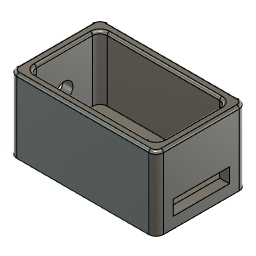
IIT Plant Watch v3 (Autodesk Fusion 360 design; units mm, degrees)
Autodesk Fusion 360 part; units mm, degrees
sketch "Sketch1" plane through (0, 0, 0) normal (0, 1, 0) x (1, 0, 0) in component "Box"
  line L0 (30, -18.5) -> (-30, -18.5)
  line L1 (-30, -18.5) -> (-30, 18.5)
  line L2 (-30, 18.5) -> (30, 18.5)
  line L3 (30, 18.5) -> (30, -18.5)
  line L4 (30, -18.5) -> (-30, 18.5) construction
  line L5 (-30, -18.5) -> (30, 18.5) construction
  dimension "d1" = 60
  dimension "d2" = 37
  constraint horizontal L0
  constraint perpendicular L0 L1
  constraint parallel L0 L2
  constraint parallel L1 L3
  constraint coincident L4 origin
  constraint coincident L5 origin
  measures "d1" distance of L1.end L2.end
  measures "d2" distance of L0.end L1.end
extrude "Extrude1" add sketch "Sketch1" along normal blind 30 in component "Box"
sketch "Sketch2" plane through (0, 30, 0) normal (0, 1, 0) x (-1, 0, 0) in component "Box"
  line L0 (-30, -18.5) -> (30, -18.5)
  line L1 (30, -18.5) -> (30, 18.5)
  line L2 (30, 18.5) -> (-30, 18.5)
  line L3 (-30, 18.5) -> (-30, -18.5)
  line L4 (26, -14.5) -> (26, 14.5)
  line L5 (26, 14.5) -> (-26, 14.5)
  line L6 (-26, 14.5) -> (-26, -14.5)
  line L7 (-26, -14.5) -> (26, -14.5)
  dimension "d5" = -4
extrude "Extrude2" cut sketch "Sketch2" against normal up to surface (26 mm away) contours L4 L5 L6 L7 in component "Box"
fillet "Fillet1" radius 3 4 edges at (26, 17, -14.5) (26, 17, 14.5) (-26, 17, -14.5) (-26, 17, 14.5) in component "Box"
fillet "Fillet2" radius 3 4 edges at (-30, 15, 18.5) (-30, 15, -18.5) (30, 15, 18.5) (30, 15, -18.5) in component "Box"
sketch "Sketch3" plane through (0, 0, 18.5) normal (0, 0, 1) x (1, 0, 0) in component "Box"
  line L0 (27, 0) -> (27, 30)
  line L1 (27, 30) -> (-27, 30)
  line L2 (-27, 30) -> (-27, 0)
  line L3 (-27, 0) -> (27, 0)
sketch "Sketch4" plane through (-30, 0, 0) normal (-1, 0, 0) x (0, 0, 1) in component "Box"
  line L0 (-15.5, 30) -> (-15.5, 0)
  line L1 (-15.5, 0) -> (15.5, 0)
  line L2 (15.5, 0) -> (15.5, 30)
  line L3 (15.5, 30) -> (-15.5, 30)
  circle A0 centre (0, 15) radius 3.5
  line L4 (-18.5, 30) -> (-18.5, 0)
  dimension "d12" = 7
  dimension "d13" = 18.5
  dimension "d14" = 15
  measures "d12" diameter of A0
  measures "d13" distance of A0.centre L4
  measures "d14" distance of L1 A0.centre
extrude "Extrude3" cut sketch "Sketch4" against normal up to surface (4 mm away) contours A0 in component "Box"
sketch "Sketch5" plane through (30, 0, 0) normal (1, 0, 0) x (0, 0, -1) in component "Box"
  line L0 (15.5, 0) -> (15.5, 30)
  line L1 (15.5, 30) -> (-15.5, 30)
  line L2 (-15.5, 30) -> (-15.5, 0)
  line L3 (-15.5, 0) -> (15.5, 0)
  line L4 (0, 0) -> (0, 36) construction
  line L5 (11.5, 4.5) -> (-11.5, 4.5)
  line L6 (-11.5, 4.5) -> (-11.5, 10.5)
  line L7 (-11.5, 10.5) -> (11.5, 10.5)
  line L8 (11.5, 10.5) -> (11.5, 4.5)
  line L9 (11.5, 4.5) -> (-11.5, 10.5) construction
  line L10 (-11.5, 4.5) -> (11.5, 10.5) construction
  point P0 (0, 7.5)
  dimension "d17" = 23
  dimension "d18" = 6
  dimension "d19" = 7.5
  constraint coincident L4.start origin
  constraint perpendicular L1 L4
  constraint horizontal L5
  constraint perpendicular L5 L6
  constraint parallel L5 L7
  constraint parallel L6 L8
  constraint coincident L9 P0
  constraint coincident L10 P0
  constraint coincident L4 P0
  measures "d17" distance of L6.end L7.end
  measures "d18" distance of L5.end L6.end
  measures "d19" distance of L3 P0
extrude "Extrude4" cut sketch "Sketch5" against normal up to surface (4 mm away) contours L5 L6 L7 L8 in component "Box"
sketch "Sketch6" plane through (0, 0, 0) normal (0, -1, 0) x (1, 0, 0) in component "Box"
  arc A0 (27, -18.5) -> (30, -15.5) centre (27, -15.5) ccw
  line L0 (30, -15.5) -> (30, 15.5)
  arc A1 (30, 15.5) -> (27, 18.5) centre (27, 15.5) ccw
  line L1 (27, 18.5) -> (-27, 18.5)
  arc A2 (-27, 18.5) -> (-30, 15.5) centre (-27, 15.5) ccw
  line L2 (-30, 15.5) -> (-30, -15.5)
  arc A3 (-30, -15.5) -> (-27, -18.5) centre (-27, -15.5) ccw
  line L3 (-27, -18.5) -> (27, -18.5)
  line L4 (-30, 0) -> (37.1551, 0) construction
  circle A4 centre (-20, 0) radius 2
  dimension "d22" = 4
  dimension "d26" = 10
  constraint midpoint L2 L4.start
  constraint perpendicular L0 L4
  constraint coincident L4 A4.centre
  measures "d22" diameter of A4
  measures "d26" distance of L2 A4.centre
extrude "Extrude5" cut sketch "Sketch6" against normal up to surface (4 mm away) contours A4 in component "Box"
fillet "Fillet4" radius 1 16 edges at (-25.1213, 30, 13.6213) (-26, 30, 0) (-25.1213, 30, -13.6213) (0, 30, -14.5) (25.1213, 30, -13.6213) (26, 30, 0) (25.1213, 30, 13.6213) (0, 30, 14.5) (-29.1213, 30, -17.6213) (-30, 30, 0) (-29.1213, 30, 17.6213) (0, 30, 18.5) (29.1213, 30, 17.6213) (30, 30, 0) (29.1213, 30, -17.6213) (0, 30, -18.5) in component "Box"
component "Box" placed x (1, 0, 0) y (0, 1, 0) z (0, 0, 1) at (0, 0, 0)
component "Lid" placed x (1, 0, 0) y (0, 1, 0) z (0, 0, 1) at (0, 0, 0)
